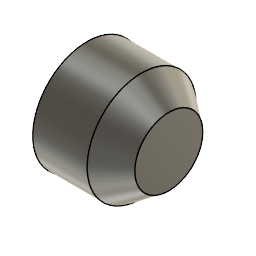
turning(fusion) (Autodesk Fusion 360 design; units mm, degrees)
part number: 2026-06-24-22-11-30-896
Autodesk Fusion 360 part; units mm, degrees
sketch "Sketch1" plane through (0, 0, 0) normal (0, 0, 1) x (1, 0, 0)
  line L0 (0, 0) -> (0, 80)
  line L1 (0, 80) -> (80, 80)
  line L2 (80, 80) -> (120, 50)
  line L3 (120, 50) -> (120, 0)
  line L4 (120, 0) -> (0, 0)
  constraint coincident L0.start L4.end
  constraint vertical L0
  constraint perpendicular L0 L1
  constraint perpendicular L1 L3
  constraint perpendicular L0 L4
revolve "Revolve1" add sketch "Sketch1" angle 360 about axis through (120, 0, 0) along (-1, 0, 0)
